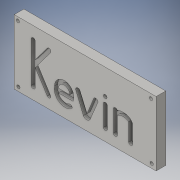
# Autodesk Inventor part: Part1
Saved by Autodesk Inventor 2016 (Build 200138000, 138)
## iProperties
Created: 2016-09-22
Part Number: Part1
Material: Generic
Document SubType Name: Modeling
Designer: Kevin G
Density: 1 g/cm^3
Appearance: Default
Author: Kevin G
Autodesk Inventor part; units mm, degrees
ref_plane "YZ Plane" through (0, 0, 0) normal (1, 0, 0) x (0, 1, 0)
ref_plane "XZ Plane" through (0, 0, 0) normal (0, 1, 0) x (-1, 0, 0)
ref_plane "XY Plane" through (0, 0, 0) normal (0, 0, 1) x (1, 0, 0)
sketch "Sketch1" plane through (0, 0, 0) normal (0, 0, 1) x (1, 0, 0)
  line L0 (-137.5833, 63.5) -> (141.8167, 63.5)
  line L1 (141.8167, 63.5) -> (141.8167, -63.5)
  line L2 (141.8167, -63.5) -> (-137.5833, -63.5)
  line L3 (-137.5833, -63.5) -> (-137.5833, 63.5)
  point P0 (0, 0)
  dimension "d0" = 127
  dimension "d1" = 279.4
  constraints: 8 end point, 2 parallel, 1 horizontal, 1 perpendicular
  measures "d0" distance of L2.end L0.start
  measures "d1" distance of L1.end L2.end
extrude "Extrusion1" add sketch "Sketch1" along normal blind 19.05
sketch "Sketch2" plane through (0, 0, 19.05) normal (0, 0, 1) x (1, 0, 0)
  line L0 (-104.11, 39.0065) -> (-104.11, -40.3685)
  line L1 (-96.1725, 39.0065) -> (-96.1725, -40.3685)
  arc A0 (-96.1725, 39.0065) -> (-104.11, 39.0065) centre (-100.1412, 39.0065) ccw
  arc A1 (-104.11, -40.3685) -> (-96.1725, -40.3685) centre (-100.1412, -40.3685) ccw
  line L2 (-96.1725, 7.2565) -> (-72.3582, 39.0089)
  line L3 (-66.0074, 34.2457) -> (-95.773, -5.4418)
  arc A2 (-66.0074, 34.2457) -> (-72.3582, 39.0089) centre (-69.1828, 36.6273) ccw
  line L4 (-95.773, -5.4418) -> (-91.0105, 0.9082)
  line L5 (-91.0105, 0.9082) -> (-66.0074, -38.7793)
  line L6 (-96.1725, -5.9726) -> (-72.4434, -42.6525)
  arc A3 (-72.4434, -42.6525) -> (-66.0074, -38.7793) centre (-69.2883, -40.6114) ccw
  line L7 (-50.2695, -18.4324) -> (-28.0445, -18.4324)
  arc A4 (-28.0445, -18.4324) -> (-50.2695, -18.4324) centre (-39.157, -18.4324) ccw
  arc A5 (-20.107, -18.4324) -> (-58.207, -18.4324) centre (-39.157, -18.4324) ccw
  line L8 (-50.2695, -26.3699) -> (-23.282, -26.3699)
  arc A6 (-21.8395, -26.3699) -> (-20.107, -18.4324) centre (-39.157, -18.4324) ccw
  line L9 (-21.8395, -26.3699) -> (-23.282, -26.3699)
  arc A7 (-58.207, -18.4324) -> (-23.282, -39.0699) centre (-37.6419, -23.5006) ccw
  arc A8 (-50.2695, -26.3699) -> (-30.7959, -35.5495) centre (-36.251, -21.8764) ccw
  arc A9 (-23.282, -39.0699) -> (-30.7959, -35.5495) centre (-27.6387, -38.5897) ccw
  line L10 (-8.7117, 0.2232) -> (5.8463, -33.6944)
  line L11 (5.8463, -33.6944) -> (19.6609, 0.4534)
  line L12 (-16.8172, -2.8361) -> (-1.4327, -40.809)
  line L13 (27.6506, -2.8368) -> (11.7736, -40.809)
  line L14 (45.8831, 0.5315) -> (45.8831, -41.2077)
  line L15 (37.9456, -41.2077) -> (37.9456, 0.5315)
  arc A10 (37.9456, -41.2077) -> (45.8831, -41.2077) centre (41.9144, -40.414) ccw
  arc A11 (45.8831, 0.5315) -> (37.9456, 0.5315) centre (41.9144, -0.4277) ccw
  circle A12 centre (41.7382, 13.4284) radius 3.5498
  line L16 (57.6132, -41.2077) -> (57.6132, 0.5315)
  arc A13 (57.6132, -41.2077) -> (65.5507, -41.2077) centre (61.5819, -40.5108) ccw
  line L17 (65.5507, -41.2077) -> (65.5507, -6.281)
  arc A14 (87.7757, -6.281) -> (65.5507, -6.281) centre (76.6632, -23.0142) ccw
  arc A15 (87.7757, 2.1517) -> (65.5507, 2.1517) centre (76.6632, -24.7519) ccw
  line L18 (87.7757, -6.281) -> (87.7757, -41.2077)
  arc A16 (87.7757, -41.2077) -> (95.7132, -41.2077) centre (91.7444, -40.6053) ccw
  line L19 (95.7132, -41.2077) -> (95.7132, -6.281)
  arc A17 (95.7132, -6.281) -> (87.7757, 2.1517) centre (81.7338, -11.4873) ccw
  arc A18 (65.5507, 0.5315) -> (57.6132, 0.5315) centre (61.5819, 0.5315) ccw
  line L20 (65.5507, 2.1517) -> (65.5507, 0.5315)
  line L21 (5.6931, -33.3375) -> (5.8463, -33.6944)
  line L22 (6.35, -32.4492) -> (7.9173, -28.575)
  line L23 (-2.5198, -38.1257) -> (-1.4327, -40.809)
  line L24 (12.8244, -38.296) -> (11.7736, -40.809)
  line L25 (9.3001, -43.2428) -> (9.3001, -43.2428)
  arc A19 (-1.5152, -40.6053) -> (11.8588, -40.6053) centre (5.1718, -36.7416) ccw
  arc A20 (-8.4324, -0.4277) -> (-16.6723, -3.1936) centre (-12.0585, -3.2818) ccw
  arc A21 (27.5014, -3.1936) -> (19.3703, -0.2649) centre (22.9247, -3.1484) ccw
  point P0 (0, 0)
  constraints: 52 end point, 43 point on circle, 22 centre point, 15 point on line, 11 tangent, 6 vertical, 2 collinear, 2 horizontal
emboss "Emboss1" sketch "Sketch2" operation cut depth 6.35 direction (0, 0, -1)
hole "Hole1" at (131.7329, 54.9658, 19.05) direction (0, 0, -1) diameter 6.35 end through all
hole "Hole2" at (133.0632, -54.8825, 19.05) direction (0, 0, -1) diameter 6.35 end through all
hole "Hole3" at (-129.1765, -55.4493, 19.05) direction (0, 0, -1) diameter 6.35 end through all
hole "Hole4" at (-130.3028, 56.5105, 19.05) direction (0, 0, -1) diameter 6.35 end through all
body "Solid1"
